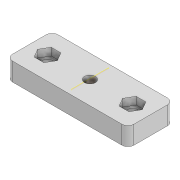
# Autodesk Inventor part: shaft pusher top
Saved by Autodesk Inventor 2020 (Build 240168000, 168)
## iProperties
Created: 2020-05-29
Part Number: shaft pusher top
Material: Generic
Document SubType Name: Modeling
Designer: mrbeh
Density: 1 g/cm^3
Appearance: Default
Author: mrbeh
Autodesk Inventor part; units mm, degrees
ref_plane "YZ Plane" through (0, 0, 0) normal (1, 0, 0) x (0, 1, 0)
ref_plane "XZ Plane" through (0, 0, 0) normal (0, 1, 0) x (-1, 0, 0)
ref_plane "XY Plane" through (0, 0, 0) normal (0, 0, 1) x (1, 0, 0)
sketch "Sketch1" plane through (0, 0, 0) normal (0, 1, 0) x (-1, 0, 0)
  line L0 (0, 0) -> (40, 0)
  line L1 (40, 0) -> (40, -15)
  line L2 (40, -15) -> (0, -15)
  line L3 (0, -15) -> (0, 0)
  dimension "d0" = 40
  dimension "d1" = 15
  constraints: 8 end point, 2 parallel, 1 horizontal, 1 perpendicular
  measures "d0" distance of L1.end L2.end
  measures "d1" distance of L0.end L1.end
extrude "Extrusion1" add sketch "Sketch1" along normal blind 6
fillet "Fillet1" radius 2 4 edges at (0, 3, 0) (0, 3, -15) (-40, 3, -15) (-40, 3, 0)
ref_plane "Work Plane1" through (-20, 0, -2) normal (1, 0, 0) x (0, 0, -1)
sketch "Sketch2" plane through (0, 6, 0) normal (0, 1, 0) x (1, 0, 0)
  circle A0 centre (-6, 7.5) radius 1.8
  point P0 (0, 0)
  dimension "d9" = 3.6
  constraints: 1 centre point
  measures "d9" diameter of A0
extrude "Extrusion3" cut sketch "Sketch2" against normal blind 6
sketch "Sketch4" plane through (0, 6, 0) normal (0, 1, 0) x (1, 0, 0)
  circle A0 centre (-6, 7.5) radius 1.8 projected
  line L0 (-7.6166, 4.7) -> (-9.2332, 7.5)
  line L1 (-9.2332, 7.5) -> (-7.6166, 10.3)
  line L2 (-7.6166, 10.3) -> (-4.3834, 10.3)
  line L3 (-4.3834, 10.3) -> (-2.7668, 7.5)
  line L4 (-2.7668, 7.5) -> (-4.3834, 4.7)
  line L5 (-4.3834, 4.7) -> (-7.6166, 4.7)
  point P0 (0, 0)
  point P1 (-6, 4.7)
  constraints: 12 end point, 1 coincident, 1 midpoint, 13 other
extrude "Extrusion4" cut sketch "Sketch4" against normal blind 2.5
sketch "Sketch5" plane through (0, 6, 0) normal (0, 1, 0) x (1, 0, 0)
  circle A0 centre (-20, 7.5) radius 1.8
  point P0 (0, 0)
  dimension "d15" = 3.6
  constraints: 1 centre point
  measures "d15" diameter of A0
extrude "Extrusion5" cut sketch "Sketch5" against normal blind 6
sketch "Sketch6" plane through (0, 0, 0) normal (0, -1, 0) x (1, 0, 0)
  circle A0 centre (-20, -7.5) radius 1.8 projected
  line L0 (-21.6166, -10.3) -> (-23.2332, -7.5)
  line L1 (-23.2332, -7.5) -> (-21.6166, -4.7)
  line L2 (-21.6166, -4.7) -> (-18.3834, -4.7)
  line L3 (-18.3834, -4.7) -> (-16.7668, -7.5)
  line L4 (-16.7668, -7.5) -> (-18.3834, -10.3)
  line L5 (-18.3834, -10.3) -> (-21.6166, -10.3)
  point P0 (0, 0)
  point P1 (-20, -10.3)
  constraints: 12 end point, 1 coincident, 1 midpoint, 13 other
extrude "Extrusion6" cut sketch "Sketch6" against normal blind 2.5
mirror "Mirror1" about plane through (-20, 0, -2) normal (1, 0, 0) of "Extrusion3"
mirror "Mirror2" about plane through (-20, 0, -2) normal (1, 0, 0) of "Extrusion4"
body "Solid1"
